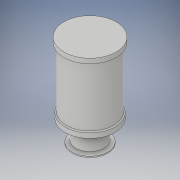
# Autodesk Inventor part: Newport SL 1200-422
Saved by Autodesk Inventor 2018 (Build 220112000, 112)
## iProperties
Created: 2018-01-29
Part Number: Newport SL 1200-422
Material: Generic
Document SubType Name: Modeling
Designer: Rich
Density: 1 g/cm^3
Appearance: Default
Author: Rich
Autodesk Inventor part; units mm, degrees
ref_plane "YZ Plane" through (0, 0, 0) normal (1, 0, 0) x (0, 1, 0)
ref_plane "XZ Plane" through (0, 0, 0) normal (0, 1, 0) x (-1, 0, 0)
ref_plane "XY Plane" through (0, 0, 0) normal (0, 0, 1) x (1, 0, 0)
sketch "Sketch1" plane through (0, 0, 0) normal (0, 0, 1) x (-1, 0, 0)
  line L0 (0, -67.1677) -> (0, 491.6323)
  line L1 (0, 491.6323) -> (-95.25, 491.6323)
  line L2 (-95.25, 491.6323) -> (-95.25, 485.2823)
  line L3 (-95.25, 485.2823) -> (-63.5, 485.2823)
  line L4 (-63.5, 485.2823) -> (-60.325, 482.1073)
  line L5 (-60.325, 482.1073) -> (-63.5308, 477.5289)
  line L6 (-63.5308, 477.5289) -> (-76.2, 477.5289)
  line L7 (-76.2, 477.5289) -> (-76.2, 375.9289)
  line L8 (-76.2, 375.9289) -> (-133.35, 375.9289)
  line L9 (-133.35, 375.9289) -> (-133.35, 350.5289)
  line L10 (-133.35, 350.5289) -> (-127, 346.0826)
  line L11 (-127, 346.0826) -> (-127, 25.4)
  line L12 (-127, 25.4) -> (-139.7, 25.4)
  line L13 (-139.7, 25.4) -> (-139.7, 0)
  line L14 (-139.7, 0) -> (0, 0)
  line L15 (0, 0) -> (0, 491.6323)
  dimension "d1" = 127
  dimension "d2" = 25.4
  dimension "d3" = 12.7
  dimension "d4" = 95.25
  dimension "d5" = 6.35
  dimension "d6" = 558.8
  dimension "d7" = 6.35
  dimension "d9" = 63.5
  dimension "d10" = 76.2
  dimension "d11" = 101.6
  dimension "d12" = 35
  dimension "d13" = 135
  dimension "d14" = 25.4
  dimension "d15" = 3.175
  constraints: 32 end point, 9 perpendicular, 2 horizontal, 1 collinear, 1 parallel, 1 vertical
  measures "d1" distance between parallel lines of L0 L11
  measures "d2" distance of L12.end L13.end
  measures "d3" distance of L11.end L12.end
  measures "d4" distance of L0.end L1.end
  measures "d5" distance of L1.end L2.end
  measures "d6" distance of L0.start L0.end
  measures "d7" distance between parallel lines of L11 L9
  measures "d9" distance from line of L0 L3.end
  measures "d10" distance between parallel lines of L0 L7
  measures "d11" distance of L6.end L7.end
  measures "d12" angle of L0 L5
  measures "d13" angle of L3 L4
  measures "d14" distance of L8.end L9.end
  measures "d15" distance from line of L3 L4.end
revolve "Revolution1" add sketch "Sketch1" angle 360 about axis through (0, 67.1677, 0) along (0, -1, 0)
body "Solid1"
